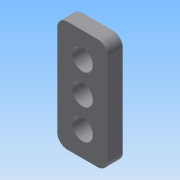
# Autodesk Inventor part: spacer
Saved by Autodesk Inventor 2015 (Build 190159000, 159)
## iProperties
Created: 2016-12-01
Part Number: spacer
Material: Générique
Document SubType Name: Modeling
Designer: Gregwar
Density: 1 g/cm^3
Appearance: Par défaut
Author: Gregwar
Autodesk Inventor part; units mm, degrees
ref_plane "YZ Plane" through (0, 0, 0) normal (1, 0, 0) x (0, 1, 0)
ref_plane "XZ Plane" through (0, 0, 0) normal (0, 1, 0) x (-1, 0, 0)
ref_plane "XY Plane" through (0, 0, 0) normal (0, 0, 1) x (1, 0, 0)
sketch "Esquisse1" plane through (0, 0, 0) normal (0, 1, 0) x (-1, 0, 0)
  line L0 (0, 0) -> (10, 0)
  line L1 (10, 0) -> (10, -22)
  line L2 (10, -22) -> (0, -22)
  line L3 (0, -22) -> (0, 0)
  line L4 (5, 0) -> (5, -22) construction
  line L5 (10, -11) -> (0, -11) construction
  circle A0 centre (5, -11) radius 2.05
  circle A1 centre (5, -17) radius 2.05
  circle A2 centre (5, -5) radius 2.05
  dimension "d0" = 4.1
  dimension "d1" = 5
  dimension "d2" = 6
  dimension "d3" = 5
  constraints: 12 end point, 5 midpoint, 3 centre point, 2 parallel, 1 equal radius, 1 horizontal, 1 perpendicular, 1 point on line, 1 symmetric about line, 1 other
  measures "d0" diameter of A1
  measures "d1" distance from line of A1.centre L2
  measures "d2" distance of A0.centre A1.centre
  measures "d3" distance from line of L1 A0.centre
extrude "Extrusion1" add sketch "Esquisse1" along normal blind 3
fillet "Congé1" radius 2 4 edges at (-10, 1.5, 0) (0, 1.5, 0) (0, 1.5, -22) (-10, 1.5, -22)
equation "\"d3\" = d1"
